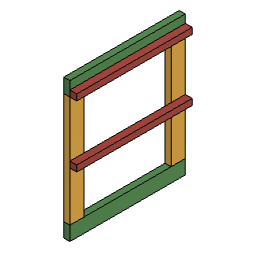
GarageStorage (Autodesk Fusion 360 design; units mm, degrees)
Autodesk Fusion 360 part; units mm, degrees
sketch "Sketch1" plane through (0, 0, 0) normal (0, 0, 1) x (1, 0, 0)
  line L0 (0, 0) -> (497.84, 0)
  line L1 (497.84, 0) -> (497.84, 723.9)
  line L2 (497.84, 723.9) -> (0, 723.9)
  line L3 (0, 723.9) -> (0, 0)
  line L4 (248.92, 723.9) -> (274.32, 723.9)
  line L5 (274.32, 723.9) -> (274.32, 0)
  line L6 (274.32, 0) -> (248.92, 0)
  line L7 (248.92, 0) -> (248.92, 723.9)
  dimension "d4" = 497.84
  dimension "d5" = 723.9
  dimension "d8" = 25.4
  dimension "d9" = 723.9
  constraint horizontal L0
  constraint vertical L1
  constraint horizontal L2
  constraint vertical L3
  constraint coincident L0.start L3.end
  constraint horizontal L4
  constraint vertical L5
  constraint horizontal L6
  constraint vertical L7
  constraint midpoint L2 L4.start
  measures "d4" distance of L0.start L0.end
  measures "d5" distance of L0.start L2.end
  measures "d8" distance of L4.start L4.end
  measures "d9" distance of L4.start L6.end
extrude "Extrude1" add sketch "Sketch1" along normal blind 25.4 makes body 1
extrude "Extrude2" add sketch "Sketch1" against normal blind 360.68 contours L0 L2 L4 L5 L6 L7 bodies 1
sketch "Sketch1 (2)" plane through (0, 0, 0) normal (0, 1, 0) x (1, 0, 0) in component "OutsideBraces"
  line L0 (0, 0) -> (38.1, 0)
  line L1 (38.1, 0) -> (38.1, -88.9)
  line L2 (38.1, -88.9) -> (0, -88.9)
  line L3 (0, -88.9) -> (0, 0)
  dimension "d20" = 38.1
  dimension "d21" = 88.9
  constraint horizontal L0
  constraint vertical L1
  constraint horizontal L2
  constraint vertical L3
  constraint coincident L0.start L3.end
  measures "d20" distance of L0.start L0.end
  measures "d21" distance of L0.start L2.end
extrude "Extrude1'" add sketch "Sketch1 (2)" along normal blind 723.9 separate body makes body 2 in component "L/R_Braces"
sketch "Sketch2" plane through (0, 0, 88.9) normal (0, 0, 1) x (-1, 0, 0) in component "OutsideBraces"
  line L0 (0, 0) -> (-38.1, 0)
  line L1 (-38.1, 0) -> (-38.1, -723.9)
  line L2 (-38.1, -723.9) -> (0, -723.9)
  line L3 (0, -723.9) -> (0, 0)
  line L4 (0, 0) -> (-38.1, 0)
  line L5 (-38.1, 0) -> (-38.1, -88.9)
  line L6 (-38.1, -88.9) -> (0, -88.9)
  line L7 (0, -88.9) -> (0, 0)
  dimension "d26" = 38.1
  dimension "d27" = 88.9
  constraint horizontal L4
  constraint vertical L5
  constraint horizontal L6
  constraint vertical L7
  constraint coincident L0.start L3.end
  measures "d26" distance of L0.start L0.end
  measures "d27" distance of L0.start L6.end
extrude "Extrude1''" add sketch "Sketch2" along normal blind 695.96 separate body contours L0 L1 L3 L4 L5 L6 L7 makes body 3 in component "T/B Braces"
sketch "Sketch3" plane through (38.1, 0, 25.4) normal (1, 0, 0) x (0, 1, 0) in component "OutsideBraces"
  line L0 (0, 848.36) -> (0, 759.46)
  line L1 (0, 759.46) -> (723.9, 759.46)
  line L2 (723.9, 759.46) -> (723.9, 848.36)
  line L3 (723.9, 848.36) -> (0, 848.36)
  line L4 (0, 797.56) -> (723.9, 797.56)
  line L5 (723.9, 797.56) -> (723.9, 759.46)
  line L6 (723.9, 759.46) -> (0, 759.46)
  line L7 (0, 759.46) -> (0, 797.56)
  line L8 (0, 398.78) -> (723.9, 398.78)
  line L9 (0, 360.68) -> (0, 398.78)
  line L10 (723.9, 360.68) -> (0, 360.68)
  line L11 (723.9, 398.78) -> (723.9, 360.68)
  point P0 (0, 797.56)
  dimension "d30" = 50.8
  dimension "d31" = 723.9
  dimension "d32" = 38.1
  dimension "d37" = 0
  constraint horizontal L4
  constraint vertical L5
  constraint horizontal L6
  constraint vertical L7
  constraint coincident P0 L4.start
  measures "d30" distance of L0.start P0
  measures "d31" distance of P0 L4.end
  measures "d32" distance of P0 L0.end
extrude "Extrude1'''" add sketch "Sketch3" along normal blind 42.8625 separate body contours L0 L1 L2 L4 L5 L6 L7 makes body 4 in component "Toat Rale"
move_body "Move1" bodies 1 to x (1, 0, 0) y (0, 1, 0) z (0, 0, 1) at (-159.2705, 0, 824.7298)
copy_body "CopyPasteBodies1" bodies 1 makes body 5
move_body "Move2" bodies 5 to x (1, 0, 0) y (0, 1, 0) z (0, 0, 1) at (40.2545, 0, -389.6638)
component "OutsideBraces" placed x (1, 0, 0) y (0, 1, 0) z (0, 0, 1) at (0, 0, 0)
component "T/B Braces" placed x (1, 0, 0) y (0, 1, 0) z (0, 0, 1) at (0, 0, 0) in component "OutsideBraces"
component "T/B Braces" placed x (1, 0, 0) y (0, 1, 0) z (0, 0, 1) at (0, 635, 0) in component "OutsideBraces"
component "L/R_Braces" placed x (1, 0, 0) y (0, 1, 0) z (0, 0, 1) at (0, 0, 0) in component "OutsideBraces"
component "L/R_Braces" placed x (1, 0, 0) y (0, 1, 0) z (0, 0, 1) at (0, 0, 784.86) in component "OutsideBraces"
component "Toat Rale" placed x (1, 0, 0) y (0, 1, 0) z (0, 0, 1) at (0, 0, 0) in component "OutsideBraces"
component "Toat Rale" placed x (1, 0, 0) y (0, 1, 0) z (0, 0, 1) at (0, 0, -386.08) in component "OutsideBraces"
equation "ST_Height = 15.2 in"
equation "ST_Width = 19.6 in"
equation "ST_Length = 28.5 in"
equation "d4 = ST_Width"
equation "d5 = ST_Length"
equation "d9 = ST_Length"
equation "d10 = -ST_Height + 1 in"
equation "blade_kerf = ( 1 / 8 ) * 1 in"
equation "Brace_thickness = 1.5 in"
equation "Brace_width = 3.5 in"
equation "ToteRale_width = ( Brace_width / 2 ) - ( blade_kerf / 2 )"
equation "ToteRale_thickness = Brace_thickness"
equation "numOfShelves = 2"
equation "SpaceBTWShelves = 2 in"
equation "Side_Height = ( ( ST_Height + SpaceBTWShelves ) * numOfShelves ) - ( Brace_width * 2 )"
equation "d20 = Brace_thickness"
equation "d21 = Brace_width"
equation "Brace_length = ST_Length"
equation "Side_length = Brace_length + 1.5 in"
equation "d24 = Brace_length"
equation "d26 = Brace_thickness"
equation "d27 = Brace_width"
equation "d28 = Side_Height"
equation "d30 = SpaceBTWShelves"
equation "d31 = Brace_length"
equation "d32 = ToteRale_thickness"
equation "d33 = ToteRale_width"
equation "d36 = numOfShelves"
equation "d38 = -ST_Height + Brace_thickness - SpaceBTWShelves"
